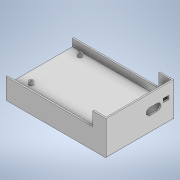
# Autodesk Inventor part: SD2104_case_design2
Saved by Autodesk Inventor 2022 (Build 260153000, 153)
## iProperties
Created: 2021-11-06
Part Number: SD2104_case_design2
Material: Generic
Document SubType Name: Modeling
Designer: Karl
Density: 1 g/cm^3
Appearance: Default
Author: Karl
Autodesk Inventor part; units mm, degrees
ref_plane "YZ Plane" through (0, 0, 0) normal (1, 0, 0) x (0, 1, 0)
ref_plane "XZ Plane" through (0, 0, 0) normal (0, 1, 0) x (-1, 0, 0)
ref_plane "XY Plane" through (0, 0, 0) normal (0, 0, 1) x (1, 0, 0)
sketch "Sketch1" plane through (0, 0, 0) normal (0, 0, 1) x (1, 0, 0)
  line L0 (-46.99, -16.0401) -> (46.99, -16.0401)
  line L1 (46.99, -16.0401) -> (46.99, 16.0401)
  line L2 (46.99, 16.0401) -> (-46.99, 16.0401)
  line L3 (-46.99, 16.0401) -> (-46.99, -16.0401)
  line L4 (-46.99, -16.0401) -> (46.99, 16.0401) construction
  line L5 (46.99, -16.0401) -> (-46.99, 16.0401) construction
  line L6 (46.99, 16.0401) -> (34.29, 16.0401)
  line L7 (34.29, 16.0401) -> (34.29, 3.3401)
  line L8 (34.29, 3.3401) -> (-46.99, 3.3401)
  point P0 (0, 0)
  dimension "d0" = 93.98
  dimension "d1" = 32.0802
  dimension "d2" = 12.7
  dimension "d3" = 12.7
  constraints: 18 end point, 2 midpoint, 2 parallel, 2 perpendicular, 2 point on line, 1 horizontal, 1 vertical
  measures "d0" distance of L2.end L1.end
  measures "d1" distance of L1.end L0.end
  measures "d2" distance of L1.end L6.end
  measures "d3" distance of L6.end L7.end
extrude "Extrusion1" add sketch "Sketch1" along normal blind 63.5 contours L3 L8 L7 L2 L1 L0
shell "Shell1" thickness 1.27 removed faces 4 at (-46.99, -3.12, 21.1667) at (7.1967, 3.3401, 21.1667) at (34.29, 11.8068, 42.3333) at (42.7567, 16.0401, 21.1667)
sketch "Sketch2" plane through (45.72, -14.7701, 1.27) normal (-1, 0, 0) x (0, 0, 1)
  line L0 (0, 0) -> (0, 8.7122)
  line L1 (0, 8.7122) -> (0, 11.2522)
  line L2 (0, 0) -> (0, 30.8102) projected
  line L3 (0, 11.2522) -> (0, 16.3322)
  line L4 (0, 18.1102) -> (0, 30.8102) projected
  line L5 (0, 16.3322) -> (0, 30.8102)
  line L6 (0, 11.2522) -> (60.96, 11.2522)
  line L7 (60.96, 18.1102) -> (60.96, 0) projected
  line L8 (60.96, 8.7122) -> (0, 8.7122)
  point P0 (-1.27, 14.7701)
  point P1 (60.96, 8.7122)
  dimension "d7" = 8.7122
  dimension "d8" = 2.54
  dimension "d9" = 5.08
  dimension "d10" = 14.478
  constraints: 12 end point, 3 point on line, 2 vertical, 1 horizontal, 1 parallel
  measures "d7" distance of L0.start L0.end
  measures "d8" distance of L0.end L1.end
  measures "d9" distance of L1.end L3.end
  measures "d10" distance of L3.end L2.end
extrude "Extrusion2" add sketch "Sketch2" along normal up to surface (92.71 mm away)
sketch "Sketch3" plane through (45.72, -3.5179, 62.23) normal (0, 1, 0) x (1, 0, 0)
  line L0 (0, 0) -> (-11.43, 0) projected
  circle A0 centre (0, 0) radius 8.255
  line L1 (0, 60.96) -> (0, 0) projected
  line L2 (0, 8.255) -> (0, 0)
  line L3 (0, 0) -> (-8.255, 0)
  line L4 (-11.43, 60.96) -> (0, 60.96) projected
  line L5 (0, 60.96) -> (-85.725, 60.96)
  line L6 (-85.725, 60.96) -> (-85.725, 3.81)
  line L7 (-85.725, 3.81) -> (0, 3.81)
  line L8 (0, 3.81) -> (0, 60.96)
  arc A1 (-5.1304, 6.4672) -> (-2.2995, 7.9283) centre (0, 0) ccw
  line L9 (0, 0) -> (-92.71, 0) projected
  line L10 (0, 8.255) -> (0, 0)
  line L11 (0, 0) -> (-8.255, 0)
  point P0 (-45.72, 62.23)
  dimension "d13" = 16.51
  dimension "d37" = 85.725
  dimension "d38" = 57.15
  constraints: 16 end point, 6 point on circle, 2 centre point, 2 collinear, 2 parallel, 2 point on line, 1 concentric, 1 horizontal, 1 perpendicular, 1 vertical
  measures "d13" diameter of A0
  measures "d37" distance of L7.end L6.end
  measures "d38" distance of L6.end L5.end
extrude "Extrusion3" cut sketch "Sketch3" against normal up to surface (2.54 mm away) contours L0 A0 L7 L1 | L7 A0 L1
sketch "Sketch4" plane through (-46.99, -3.5179, 1.27) normal (0, 1, 0) x (1, 0, 0)
  line L0 (93.98, 1.27) -> (93.98, -62.23) projected
  line L1 (92.71, 0) -> (6.985, 0)
  line L2 (6.985, 0) -> (6.985, -53.975)
  line L3 (6.985, -53.975) -> (92.71, -53.975)
  line L4 (92.71, -53.975) -> (92.71, 0)
  circle A0 centre (87.63, -3.048) radius 1.0287
  circle A1 centre (88.646, -49.911) radius 1.0287
  circle A2 centre (11.049, -49.911) radius 1.0287
  circle A3 centre (11.049, -4.064) radius 1.0287
  circle A4 centre (11.049, -4.064) radius 2.0193
  circle A5 centre (11.049, -49.911) radius 2.0193
  circle A6 centre (87.63, -3.048) radius 2.0193
  circle A7 centre (88.646, -49.911) radius 2.0193
  point P0 (46.99, 1.27)
  dimension "d19" = 85.725
  dimension "d20" = 53.975
  dimension "d21" = 3.048
  dimension "d22" = 5.08
  dimension "d23" = 4.064
  dimension "d24" = 4.064
  dimension "d25" = 4.064
  dimension "d26" = 4.064
  dimension "d27" = 4.064
  dimension "d28" = 4.064
  dimension "d29" = 2.0574
  dimension "d30" = 2.0574
  dimension "d31" = 2.0574
  dimension "d32" = 2.0574
  dimension "d33" = 4.0386
  dimension "d34" = 4.0386
  dimension "d35" = 4.0386
  dimension "d36" = 4.0386
  constraints: 8 centre point, 8 coincident, 8 end point, 2 parallel, 1 horizontal, 1 perpendicular
  measures "d19" distance of L3.end L2.end
  measures "d20" distance of L2.end L1.end
  measures "d21" distance from line of L1 point (87.63, -3.048)
  measures "d22" distance from line of L4 point (87.63, -3.048)
  measures "d23" distance from line of L4 point (88.646, -49.911)
  measures "d24" distance from line of L3 point (88.646, -49.911)
  measures "d25" distance from line of L3 point (11.049, -49.911)
  measures "d26" distance from line of L2 point (11.049, -49.911)
  measures "d27" distance from line of L2 point (11.049, -4.064)
  measures "d28" distance from line of L1 point (11.049, -4.064)
  measures "d29" diameter of A0
  measures "d30" diameter of A1
  measures "d31" diameter of A2
  measures "d32" diameter of A3
  measures "d33" diameter of A4
  measures "d34" diameter of A5
  measures "d35" diameter of A6
  measures "d36" diameter of A7
extrude "Extrusion4" add sketch "Sketch4" along normal blind 2.54 contours A4 | A5 | A6 | A7
sketch "Sketch5" plane through (-46.99, -3.5179, 1.27) normal (0, 1, 0) x (1, 0, 0)
  circle A0 centre (11.049, -4.064) radius 1.0287 projected
  circle A1 centre (87.63, -3.048) radius 1.0287 projected
  circle A2 centre (88.646, -49.911) radius 1.0287 projected
  circle A3 centre (11.049, -49.911) radius 1.0287 projected
  point P0 (46.99, 1.27)
  constraints: 4 coincident
extrude "Extrusion5" cut sketch "Sketch5" against normal blind 2.54
sketch "Sketch6" plane through (45.72, -14.7701, 62.23) normal (-1, 0, 0) x (0, 0, 1)
  line L0 (-57.4548, 17.2339) -> (-52.3748, 17.2339)
  line L1 (-52.3748, 17.2339) -> (-52.3748, 20.5105)
  line L2 (-52.3748, 20.5105) -> (-57.4548, 20.5105)
  line L3 (-57.4548, 20.5105) -> (-57.4548, 17.2339)
  line L4 (-57.4548, 17.2339) -> (-52.3748, 20.5105) construction
  line L5 (-52.3748, 17.2339) -> (-57.4548, 20.5105) construction
  line L6 (-54.8767, 13.7922) -> (-58.9153, 13.7922) projected
  line L7 (-62.23, 30.8102) -> (-62.23, 18.1102) projected
  line L8 (-62.23, 18.1102) -> (-62.23, -1.27) projected
  line L9 (-43.18, 13.081) -> (-39.5859, 13.081)
  line L10 (-43.18, 13.081) -> (-46.7741, 13.081)
  line L11 (-46.7741, 19.431) -> (-39.5859, 19.431)
  arc A0 (-46.7741, 19.431) -> (-46.7741, 13.081) centre (-46.7741, 16.256) ccw
  arc A1 (-39.5859, 13.081) -> (-39.5859, 19.431) centre (-39.5859, 16.256) ccw
  point P0 (-62.23, 14.7701)
  point P1 (-54.9148, 18.8722)
  point P2 (-43.18, 16.256)
  dimension "d46" = 5.08
  dimension "d47" = 3.2766
  dimension "d48" = 5.08
  dimension "d49" = 7.3152
  dimension "d62" = 19.05
  dimension "d63" = 2.4638
  dimension "d65" = 3.5941
  dimension "d66" = 3.5941
  constraints: 18 end point, 4 point on circle, 4 tangent, 3 horizontal, 2 centre point, 2 midpoint, 2 parallel, 1 perpendicular
  measures "d46" distance of L2.end L1.end
  measures "d47" distance of L1.end L0.end
  measures "d48" distance from line of point (-54.915, 18.872) L6
  measures "d49" distance from line of L7 point (-54.915, 18.872)
  measures "d62" distance from line of L8 point (-43.18, 16.256)
  measures "d63" distance from line of L6 point (-43.18, 16.256)
  measures "d65" distance of L9.start L9.end
  measures "d66" distance of L9.start L10.end
extrude "Extrusion6" cut sketch "Sketch6" against normal up to surface (1.27 mm away)
fillet "Fillet1" radius 0.635 1 edges at (46.99, -16.0401, 31.75)
body "Solid1"
